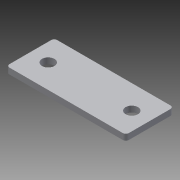
# Autodesk Inventor part: Wheel Mount Support Plate
Saved by Autodesk Inventor 2013 (Build 170138000, 138)
## iProperties
Created: 2013-01-23
Part Number: Wheel Mount Support Plate
Material: Aluminum 6061
Document SubType Name: Modeling
Designer: Moses
Mass: 13.2697 g
Surface Area: 37.7207 cm^2
Volume: 4.89658 cm^3
Density: 2.71 g/cm^3
Author: Moses
Autodesk Inventor part; units mm, degrees
ref_plane "YZ Plane" through (0, 0, 0) normal (1, 0, 0) x (0, 1, 0)
ref_plane "XZ Plane" through (0, 0, 0) normal (0, 1, 0) x (-1, 0, 0)
ref_plane "XY Plane" through (0, 0, 0) normal (0, 0, 1) x (1, 0, 0)
sketch "Sketch1" plane through (0, 0, 0) normal (0, 1, 0) x (-1, 0, 0)
  line L0 (0, 0) -> (63.5, 0)
  line L1 (63.5, 0) -> (63.5, 25.4)
  line L2 (63.5, 25.4) -> (0, 25.4)
  line L3 (0, 25.4) -> (0, 0)
  circle A0 centre (9.525, 12.7) radius 3.302
  circle A1 centre (53.975, 12.7) radius 3.302
  line L4 (9.525, 12.7) -> (53.975, 12.7) construction
  line L5 (31.75, 25.4) -> (31.75, 0) construction
  point P0 (31.75, 12.7)
  dimension "d0" = 63.5
  dimension "d2" = 25.4
  dimension "d3" = 44.45
  dimension "d4" = 6.604
  constraints: 12 end point, 4 midpoint, 2 centre point, 2 parallel, 2 perpendicular, 1 equal radius, 1 horizontal
  measures "d0" distance of L1.end L2.end
  measures "d2" distance of L0.end L1.end
  measures "d3" distance of L4.end L4.start
  measures "d4" diameter of A0
extrude "Extrusion1" add sketch "Sketch1" along normal blind 3.175
fillet "Fillet1" radius 1.5875 4 edges at (0, 1.5875, 25.4) (0, 1.5875, 0) (-63.5, 1.5875, 0) (-63.5, 1.5875, 25.4)
body "Solid1"
